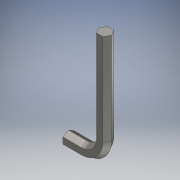
# Autodesk Inventor part: 1420-12 Cle btr-04
Saved by Autodesk Inventor 2017 (Build 210142000, 142)
## iProperties
Company: FABLAB Frenchmakers
Part Number: 1420-12 Cle btr-04
Project: 1420 VAUBAN 3D XL
Material: Acier inoxydable
Catalog Web Link: http://www.frenchmakers.com/
Document SubType Name: Modeling
Designer: Adrien MARY
Density: 8 g/cm^3
Appearance: Semi-poli
Mass: 2.36034 g
Surface Area: 4.08979 cm^2
Volume: 0.295043 cm^3
Author: Adrien MARY
Autodesk Inventor part; units mm, degrees
ref_plane "YZ Plane" through (0, 0, 0) normal (1, 0, 0) x (0, 1, 0)
ref_plane "XZ Plane" through (0, 0, 0) normal (0, 1, 0) x (-1, 0, 0)
ref_plane "XY Plane" through (0, 0, 0) normal (0, 0, 1) x (1, 0, 0)
sketch "Esquisse1" plane through (0, 0, 0) normal (0, 0, 1) x (1, 0, 0)
  line L0 (0.866, -1.5) -> (-0.866, -1.5)
  line L1 (-0.866, -1.5) -> (-1.7321, 0)
  line L2 (-1.7321, 0) -> (-0.866, 1.5)
  line L3 (-0.866, 1.5) -> (0.866, 1.5)
  line L4 (0.866, 1.5) -> (1.7321, 0)
  line L5 (1.7321, 0) -> (0.866, -1.5)
  point P0 (0, 0)
  point P1 (0, 0)
  dimension "Taille" = 3
  constraints: 12 end point, 1 coincident, 1 horizontal, 13 other
  measures "Taille" distance between parallel lines of L3 L0
sketch "Esquisse2" plane through (0, 0, 0) normal (0, 1, 0) x (-1, 0, 0)
  line L0 (0, 0) -> (0, -25)
  line L1 (5, -30) -> (10, -30)
  arc A0 (0, -25) -> (5, -30) centre (5, -25) ccw
  point P0 (0, -30)
  dimension "Grand_longueur" = 30
  dimension "Petites_longueur" = 10
  dimension "COngé" = 5
  constraints: 4 end point, 2 point on circle, 2 point on line, 2 tangent, 1 centre point, 1 perpendicular, 1 vertical
  measures "Grand_longueur" distance of L0.start point (0, -30)
  measures "Petites_longueur" distance of point (0, -30) L1.end
  measures "COngé" radius of A0
sweep "Balayage1" add profiles "Esquisse1" path "Esquisse2"
equation "\"Grand_longueur\" = 10 * Taille"
equation "\"Petites_longueur\" = 0.333333 * Grand_longueur"
